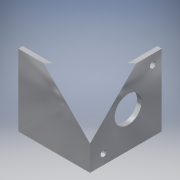
# Autodesk Inventor part: BAG motor bracket
Saved by Autodesk Inventor 2016 (Build 200138000, 138)
## iProperties
Created: 2016-01-17
Part Number: BAG motor bracket
Material: Aluminum 6061
Document SubType Name: Modeling
Designer: gus
Density: 2.7 g/cm^3
Appearance: Aluminum - Flat
Mass: 40.1967 g
Surface Area: 105.967 cm^2
Volume: 14.8876 cm^3
Author: gus
Autodesk Inventor part; units mm, degrees
ref_plane "YZ Plane" through (0, 0, 0) normal (1, 0, 0) x (0, 1, 0)
ref_plane "XZ Plane" through (0, 0, 0) normal (0, 1, 0) x (-1, 0, 0)
ref_plane "XY Plane" through (0, 0, 0) normal (0, 0, 1) x (1, 0, 0)
sketch "Sketch1" plane through (0, 0, 0) normal (0, 1, 0) x (-1, 0, 0)
  line L0 (0, 0) -> (0, 50.8)
  line L1 (0, 50.8) -> (50.8, 50.8)
  line L2 (50.8, 50.8) -> (50.8, 47.625)
  line L3 (50.8, 47.625) -> (3.175, 47.625)
  line L4 (3.175, 47.625) -> (3.175, 0)
  line L5 (3.175, 0) -> (0, 0)
  dimension "d0" = 50.8
  dimension "d1" = 50.8
  dimension "d2" = 3.175
  dimension "d3" = 47.625
  dimension "d4" = 47.625
  constraints: 12 end point, 4 perpendicular, 1 vertical
  measures "d0" distance of L0.start L0.end
  measures "d1" distance of L0.end L1.end
  measures "d2" distance of L1.end L2.end
  measures "d3" distance of L2.end L3.end
  measures "d4" distance of L3.end L4.end
extrude "Extrusion1" add sketch "Sketch1" along normal blind 50.8
sketch "Sketch3" plane through (-3.175, 0, 0) normal (-1, 0, 0) x (0, 0, 1)
  circle A0 centre (23.8125, 25.4) radius 25.4 construction
  line L0 (0, 50.8) -> (47.625, 50.8) projected
  line L1 (0, 0) -> (0, 50.8) projected
  circle A1 centre (6.3119, 43.8089) radius 2.032
  circle A2 centre (41.3131, 6.9911) radius 2.032
  line L2 (0, 0) -> (50.8, 0) projected
  line L3 (23.8125, 0) -> (23.8125, 50.8) construction
  line L4 (50.8, 50.8) -> (0, 50.8) projected
  circle A3 centre (23.8125, 25.4) radius 9.525
  dimension "d12" = 50.8
  dimension "d13" = 25.4
  dimension "d14" = 23.8125
  dimension "d15" = 4.064
  dimension "d16" = 4.064
  dimension "d17" = 17.5006
  dimension "d18" = 17.5006
  dimension "d19" = 19.05
  constraints: 4 centre point, 4 point on circle, 2 end point, 2 point on line, 1 coincident
  measures "d12" diameter of A0
  measures "d13" distance from line of A0.centre L0
  measures "d14" distance from line of L1 A0.centre
  measures "d15" diameter of A1
  measures "d16" diameter of A2
  measures "d17" distance from line of A2.centre L3
  measures "d18" distance from line of A1.centre L3
  measures "d19" diameter of A3
extrude "Extrusion2" cut sketch "Sketch3" against normal blind 3.175
body "Solid1"
